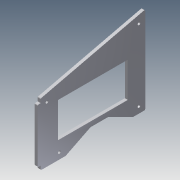
# Autodesk Inventor part: BottomRightSide
Saved by Autodesk Inventor 2014 (Build 180170000, 170)
## iProperties
Created: 2015-01-19
Part Number: BottomRightSide
Material: Generic
Document SubType Name: Modeling
Designer: Peele
Density: 1 g/cm^3
Appearance: White
Author: Peele
Autodesk Inventor part; units mm, degrees
ref_plane "YZ Plane" through (0, 0, 0) normal (1, 0, 0) x (0, 1, 0)
ref_plane "XZ Plane" through (0, 0, 0) normal (0, 1, 0) x (-1, 0, 0)
ref_plane "XY Plane" through (0, 0, 0) normal (0, 0, 1) x (1, 0, 0)
sketch "Sketch1" plane through (0, 0, 0) normal (1, 0, 0) x (0, 1, 0)
  line L0 (-105, -75) -> (105, -75)
  line L1 (105, -75) -> (105, 75)
  line L2 (105, 75) -> (-105, 75)
  line L3 (-105, 75) -> (-105, -75)
  line L4 (-105, -75) -> (105, 75) construction
  line L5 (105, -75) -> (-105, 75) construction
  point P0 (0, 0)
  point P1 (0, 0)
  point P2 (0, 0)
  dimension "d0" = 150
  dimension "d1" = 210
  constraints: 12 end point, 3 midpoint, 2 parallel, 1 coincident, 1 horizontal, 1 perpendicular
  measures "d0" distance of L2.end L0.start
  measures "d1" distance of L1.end L2.end
extrude "Extrusion1" add sketch "Sketch1" along normal blind 6
sketch "Sketch2" plane through (6, 0, 0) normal (1, 0, 0) x (0, 0, -1)
  line L0 (75, -105) -> (75, 105) projected
  line L1 (-75, -105) -> (75, -105) projected
  line L2 (75, 105) -> (100, 105)
  line L3 (100, 105) -> (100, 80)
  line L4 (100, 80) -> (75, 30)
  line L5 (75, 30) -> (75, 105)
  line L6 (75, -105) -> (75, -5)
  line L7 (75, -5) -> (100, -55)
  line L8 (100, -55) -> (100, -105)
  line L9 (100, -105) -> (75, -105)
  point P0 (0, 0)
  dimension "d4" = 25
  dimension "d5" = 50
  dimension "d25" = 50
  constraints: 16 end point, 3 equal length, 2 parallel, 2 point on line, 1 collinear, 1 horizontal, 1 perpendicular
  measures "d4" distance of L0.end L2.end
  measures "d5" vertical distance of L3.end L4.end
  measures "d25" distance of L7.end L8.end
extrude "Extrusion2" add sketch "Sketch2" against normal blind 6
sketch "Sketch3" plane through (6, 0, 0) normal (1, 0, 0) x (0, 0, -1)
  line L0 (-75, 105) -> (-75, -105) projected
  line L1 (-75, -105) -> (100, -105) projected
  line L2 (100, -105) -> (100, -55) projected
  line L3 (-75, 105) -> (-25, -105)
  line L4 (-25, -105) -> (-75, -105)
  line L5 (-75, -105) -> (-75, 105)
  point P0 (0, 0)
  dimension "d8" = 50
  constraints: 6 end point, 2 perpendicular, 1 point on line
  measures "d8" distance from line of L0 L3.end
extrude "Extrusion3" cut sketch "Sketch3" against normal through all
sketch "Sketch4" plane through (6, 0, 0) normal (1, 0, 0) x (0, 0, -1)
  line L0 (-25, -105) -> (100, -105) projected
  line L1 (100, -105) -> (100, -55) projected
  line L2 (-16.9, -105) -> (91.9, -105)
  line L3 (91.9, -105) -> (91.9, -111)
  line L4 (91.9, -111) -> (-16.9, -111)
  line L5 (-16.9, -111) -> (-16.9, -105)
  point P0 (0, 0)
  dimension "d11" = 8.1
  dimension "d12" = 8.1
  dimension "d13" = 6
  constraints: 8 end point, 2 parallel, 1 horizontal, 1 perpendicular, 1 point on line
  measures "d11" distance between parallel lines of L3 L1
  measures "d12" distance from line of L0.start L5
  measures "d13" distance between parallel lines of L0 L4
extrude "Extrusion4" add sketch "Sketch4" against normal blind 6
sketch "Sketch5" plane through (6, 0, 0) normal (1, 0, 0) x (0, 0, -1)
  line L0 (-75, 105) -> (-25, -105) projected
  line L1 (91.9, -105) -> (100, -105) projected
  line L2 (100, 80) -> (100, 105) projected
  line L3 (100, 105) -> (-75, 105) projected
  circle A0 centre (-12.5, -92.5) radius 2.7
  circle A1 centre (87.5, -67.5) radius 2.7
  circle A2 centre (87.5, 92.5) radius 2.7
  circle A3 centre (-56.5476, 92.5) radius 2.7
  line L4 (-12.5, -92.5) -> (-56.5476, 92.5) construction
  line L5 (-25, -105) -> (-16.9, -105) projected
  point P0 (0, 0)
  dimension "d17" = 12.5
  dimension "d18" = 12.5
  dimension "d19" = 12.5
  dimension "d21" = 5.4
  dimension "d22" = 37.5
  dimension "d26" = 12.5
  constraints: 4 centre point, 3 equal radius, 2 end point, 1 horizontal alignment, 1 parallel, 1 vertical alignment
  measures "d17" distance from line of A2.centre L2
  measures "d18" distance from line of A2.centre L3
  measures "d19" horizontal distance of L4.start L0.end
  measures "d21" diameter of A1
  measures "d22" distance from line of A1.centre L1
  measures "d26" distance from line of L4.start L5
extrude "Extrusion5" cut sketch "Sketch5" against normal through all
fillet "Fillet1" radius 2 10 edges at (3, -111, 16.9) (3, -105, 25) (3, -111, -91.9) (3, -105, -100) (3, 105, 75) (3, 105, -100) (3, 80, -100) (3, 30, -75) (3, -5, -75) (3, -55, -100)
sketch "Sketch6" plane through (6, 0, 0) normal (1, 0, 0) x (0, 0, -1)
  line L0 (75, -4.5279) -> (75, 29.5279) projected
  line L1 (98, 105) -> (-72.4679, 105) projected
  line L2 (91.9, -105) -> (98, -105) projected
  line L3 (-5, 70) -> (65, 70)
  line L4 (65, 70) -> (65, -70)
  line L5 (65, -70) -> (-5, -70)
  line L6 (-5, -70) -> (-5, 70)
  point P0 (0, 0)
  dimension "d27" = 10
  dimension "d28" = 35
  dimension "d29" = 35
  dimension "d30" = 70
  constraints: 8 end point, 2 parallel, 1 horizontal, 1 perpendicular
  measures "d27" distance between parallel lines of L4 L0
  measures "d28" distance between parallel lines of L3 L1
  measures "d29" distance between parallel lines of L2 L5
  measures "d30" distance of L3.start L3.end
extrude "Extrusion6" cut sketch "Sketch6" against normal through all
body "Solid1"
